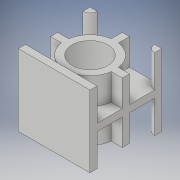
# Autodesk Inventor part: Bent beam base-120
Saved by Autodesk Inventor 2019.3 (Build 233278000, 278)
## iProperties
Created: 2019-01-29
Part Number: Bent beam base-120
Material: Generic
Document SubType Name: Modeling
Designer: Varga Daniel
Density: 1 g/cm^3
Appearance: Default
Hole_height: 8,400 mm
Beam_angle: 120,00 deg
First_hole_pos: 5,000 mm
Author: Varga Daniel
Autodesk Inventor part; units mm, degrees
ref_plane "YZ Plane" through (0, 0, 0) normal (1, 0, 0) x (0, 1, 0)
ref_plane "XZ Plane" through (0, 0, 0) normal (0, 1, 0) x (-1, 0, 0)
ref_plane "XY Plane" through (0, 0, 0) normal (0, 0, 1) x (1, 0, 0)
derived "Base_part.ipt"
sketch "Beam_sketch" plane through (0, 0, 0) normal (0, 1, 0) x (-1, 0, 0)
  line L0 (5, 0) -> (25, 0)
  line L1 (30, 5) -> (30, 25)
  line L2 (25, 30) -> (5, 30)
  line L3 (0, 25) -> (0, 5)
  line L4 (5, 29) -> (25, 29)
  line L5 (29, 25) -> (29, 5)
  line L6 (25, 1) -> (5, 1)
  line L7 (1, 5) -> (1, 25)
  circle A0 centre (5, 5) radius 2.5
  circle A1 centre (5, 5) radius 3.5
  arc A2 (25, 0) -> (30, 5) centre (25, 5) ccw
  arc A3 (30, 25) -> (25, 30) centre (25, 25) ccw
  arc A4 (5, 30) -> (0, 25) centre (5, 25) ccw
  arc A5 (0, 5) -> (5, 0) centre (5, 5) ccw
  arc A6 (1, 5) -> (5, 1) centre (5, 5) ccw
  arc A7 (5, 29) -> (1, 25) centre (5, 25) ccw
  arc A8 (29, 25) -> (25, 29) centre (25, 25) ccw
  arc A9 (25, 1) -> (29, 5) centre (25, 5) ccw
  line L8 (49.1041, 15) -> (-27.081, 15) construction
  line L9 (31.1478, 10) -> (-2.4877, 10) construction
  line L10 (-2.8604, 5) -> (35.495, 5) construction
  line L11 (5, -2.5736) -> (5, 36.7522) construction
  line L12 (15, -1.4978) -> (15, 34.8784) construction
  line L13 (1.5359, 5.5) -> (1, 5.5)
  line L14 (1.5359, 4.5) -> (1.0314, 4.5)
  line L15 (28.9686, 4.5) -> (8.4641, 4.5)
  line L16 (29, 5.5) -> (8.4641, 5.5)
  line L17 (4.5, 1.5359) -> (4.5, 1.0314)
  line L18 (5.5, 1.5359) -> (5.5, 1)
  line L19 (29, 10.5) -> (1, 10.5)
  line L20 (29, 9.5) -> (1, 9.5)
  line L21 (4.5, 28.9686) -> (4.5, 10.5)
  line L22 (4.5, 9.5) -> (4.5, 8.4641)
  line L23 (5.5, 29) -> (5.5, 10.5)
  line L24 (5.5, 9.5) -> (5.5, 8.4641)
  point P0 (0, 0)
  point P1 (30, 30)
  point P2 (0, 30)
sketch "Sketch2" plane through (0, 0, 0) normal (0, 1, 0) x (-1, 0, 0)
  circle A0 centre (0, -4) radius 2.5
  arc A1 (-1.9361, -1.0843) -> (-1.6456, -0.911) centre (0, -4) ccw
  circle A2 centre (5, 5) radius 2.5 construction
  circle A3 centre (5, 5) radius 3.5 construction
  arc A4 (-2.1242, -1.2184) -> (-1.9361, -1.0843) centre (0, -4) ccw
  circle A5 centre (0, -4) radius 3.5
  line L0 (9.2761, 0) -> (-6.9818, 0) construction
  line L1 (0, 4.8106) -> (0, -6.1444) construction
  line L2 (5, 1) -> (-5, 1)
  line L3 (5, 1) -> (5, -9)
  line L4 (5, -9) -> (-5, -9)
  line L5 (5, 0) -> (-5, 0)
  line L6 (-5, -9) -> (-5, 1)
  arc A6 (5, -8) -> (4, -9) centre (5, -9) ccw
  arc A7 (-4, -9) -> (-5, -8) centre (-5, -9) ccw
  line L7 (5, -4) -> (-5, -4) construction
  line L8 (3.4641, -4.5) -> (5, -4.5)
  line L9 (3.4641, -3.5) -> (5, -3.5)
  line L10 (-3.4641, -3.5) -> (-5, -3.5)
  line L11 (-3.4641, -4.5) -> (-5, -4.5)
  line L12 (0.5, -0.5359) -> (0.5, 0)
  line L13 (-0.5, -0.5359) -> (-0.5, 0)
  line L14 (0.5, -9) -> (0.5, -7.4641)
  line L15 (-0.5, -7.4641) -> (-0.5, -9)
  point P0 (0, 0)
  dimension "d18" = 5
  dimension "d19" = 7
  dimension "d105" = 5
  dimension "d106" = 7
  dimension "d127" = 5
  dimension "d128" = 5
  dimension "d129" = 4
  dimension "d130" = 10
  dimension "d131" = 1
  dimension "d132" = 1
  dimension "d133" = 1
  dimension "d134" = 1
  dimension "d135" = 1
  constraints: 32 end point, 17 point on line, 8 point on circle, 5 centre point, 5 collinear, 5 parallel, 4 perpendicular, 3 coincident, 3 midpoint, 2 vertical, 1 horizontal, 14 other
  measures "d18" diameter of A0
  measures "d19" diameter of A1
  measures "d105" diameter of A2
  measures "d106" diameter of A3
  measures "d127" distance between parallel lines of L3 L1
  measures "d128" distance between parallel lines of L6 L1
  measures "d129" distance from line of A0.centre L5
  measures "d130" distance between parallel lines of L4 L2
  measures "d131" distance between parallel lines of L5 L2
  measures "d132" radius of A6
  measures "d133" radius of A7
  measures "d134" distance between parallel lines of L9 L8
  measures "d135" distance between parallel lines of L13 L12
ref_plane "Work Plane2" through (-5, 0, 1) normal (0, 1, 0) x (1, 0, 0)
extrude "Extrusion16" add sketch "Sketch2" along normal mid plane 1 contours A1 L10 L6 L5 L13 A4 | A1 L15 L4 A7 L6 L11 | L12 L5 L3 L9 A1 | A1 L8 L3 A6 L4 L14
extrude "Extrusion17" add sketch "Sketch2" along normal mid plane 10 contours L5 L6 L2 L3 | A7 L4 L6 | A6 L3 L4
extrude "Extrusion18" add sketch "Sketch2" along normal mid plane 8.4 contours A4 A1 | A1 L11 L6 L10 | L13 L5 L12 A1 | A1 L14 L4 L15 | L9 L3 L8 A1
ref_plane "Work Plane3" through (0, -5, 1) normal (1, 0, 0) x (0, 0, -1)
equation "\"Beam_angle\" = 120deg"
equation "\"First_hole_pos\" = 5"
body "Solid4"
